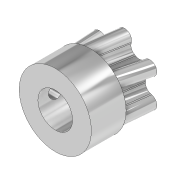
# Autodesk Inventor part: 5th Axis Drive Gear
Saved by Autodesk Inventor 2020 (Build 240168000, 168)
## iProperties
Created: 2021-06-28
Part Number: 5th Axis Drive Gear
Material: Generic
Document SubType Name: Modeling
Designer: Coy
Density: 1 g/cm^3
Appearance: Chrome - Polished
Author: Coy
Autodesk Inventor part; units mm, degrees
ref_plane "YZ Plane" through (0, 0, 0) normal (1, 0, 0) x (0, 1, 0)
ref_plane "XZ Plane" through (0, 0, 0) normal (0, 1, 0) x (-1, 0, 0)
ref_plane "XY Plane" through (0, 0, 0) normal (0, 0, 1) x (1, 0, 0)
sketch "Sketch1" plane through (0, 0, 0) normal (0, 0, 1) x (1, 0, 0)
  circle A0 centre (0, 0) radius 2.5
  circle A1 centre (0, 0) radius 5.2 construction
  line L0 (0, 0) -> (0, 5.5836) construction
  arc A2 (0.9712, 3.9619) -> (-0.9712, 3.9619) centre (0, 4.2) ccw
  line L1 (0.9221, 3.7616) -> (0.9712, 3.9619)
  line L2 (-0.9221, 3.7616) -> (-0.9712, 3.9619)
  arc A3 (-1.42, 2.6426) -> (-0.9221, 3.7616) centre (-1.8934, 3.5235) ccw
  arc A4 (0.9221, 3.7616) -> (1.42, 2.6426) centre (1.8934, 3.5235) ccw
  arc A5 (-2.9455, 2.8221) -> (-3.9167, 1.1398) centre (-3.6373, 2.1) ccw
  line L3 (-3.7187, 1.0822) -> (-3.9167, 1.1398)
  arc A6 (-2.9986, 0.0915) -> (-3.7187, 1.0822) centre (-3.9981, 0.122) ccw
  line L4 (-2.7966, 2.6794) -> (-2.9455, 2.8221)
  arc A7 (-2.7966, 2.6794) -> (-1.5786, 2.5511) centre (-2.1048, 3.4015) ccw
  arc A8 (-3.9167, -1.1398) -> (-2.9455, -2.8221) centre (-3.6373, -2.1) ccw
  line L5 (-2.7966, -2.6794) -> (-2.9455, -2.8221)
  arc A9 (-1.5786, -2.5511) -> (-2.7966, -2.6794) centre (-2.1048, -3.4015) ccw
  line L6 (-3.7187, -1.0822) -> (-3.9167, -1.1398)
  arc A10 (-3.7187, -1.0822) -> (-2.9986, -0.0915) centre (-3.9981, -0.122) ccw
  arc A11 (-0.9712, -3.9619) -> (0.9712, -3.9619) centre (0, -4.2) ccw
  line L7 (0.9221, -3.7616) -> (0.9712, -3.9619)
  arc A12 (1.42, -2.6426) -> (0.9221, -3.7616) centre (1.8934, -3.5235) ccw
  line L8 (-0.9221, -3.7616) -> (-0.9712, -3.9619)
  arc A13 (-0.9221, -3.7616) -> (-1.42, -2.6426) centre (-1.8934, -3.5235) ccw
  arc A14 (2.9455, -2.8221) -> (3.9167, -1.1398) centre (3.6373, -2.1) ccw
  line L9 (3.7187, -1.0822) -> (3.9167, -1.1398)
  arc A15 (2.9986, -0.0915) -> (3.7187, -1.0822) centre (3.9981, -0.122) ccw
  line L10 (2.7966, -2.6794) -> (2.9455, -2.8221)
  arc A16 (2.7966, -2.6794) -> (1.5786, -2.5511) centre (2.1048, -3.4015) ccw
  arc A17 (3.9167, 1.1398) -> (2.9455, 2.8221) centre (3.6373, 2.1) ccw
  line L11 (2.7966, 2.6794) -> (2.9455, 2.8221)
  arc A18 (1.5786, 2.5511) -> (2.7966, 2.6794) centre (2.1048, 3.4015) ccw
  line L12 (3.7187, 1.0822) -> (3.9167, 1.1398)
  arc A19 (3.7187, 1.0822) -> (2.9986, 0.0915) centre (3.9981, 0.122) ccw
  arc A20 (-1.42, 2.6426) -> (-1.5786, 2.5511) centre (0, 0) ccw
  arc A21 (1.5786, 2.5511) -> (1.42, 2.6426) centre (0, 0) ccw
  arc A22 (2.9986, -0.0915) -> (2.9986, 0.0915) centre (0, 0) ccw
  arc A23 (1.42, -2.6426) -> (1.5786, -2.5511) centre (0, 0) ccw
  arc A24 (-2.9986, 0.0915) -> (-2.9986, -0.0915) centre (0, 0) ccw
  arc A25 (-1.5786, -2.5511) -> (-1.42, -2.6426) centre (0, 0) ccw
  dimension "d0" = 5
  dimension "d1" = 10.4
  dimension "d3" = 2
  dimension "d4" = 2
  dimension "d5" = 2
  dimension "d8" = 360
  constraints: 48 point on circle, 26 centre point, 26 end point, 12 line through centre, 5 tangent, 2 coincident, 1 point on line, 1 vertical, 85 other
  measures "d0" diameter of A0
  measures "d1" diameter of A1
  measures "d3" diameter of A2
  measures "d4" diameter of A3
  measures "d5" diameter of A4
sketch3d "3D Sketch1"
  helix H0 starts at (2.9958, -0.0914, 0) axis through (0, 0, 0) along (0, 0, 1) pitch 166.6667 turns 0.03 hand right
sweep "Sweep1" add profiles "Sketch1" path "3D Sketch1"
sketch "Sketch2" plane through (0.787, -4.1256, 5) normal (0, 0, 1) x (0.9822873, 0.1873813, 0)
  circle A0 centre (0, 4.2) radius 2.5 projected
  arc A1 (-1.42, 6.8426) -> (-1.5786, 6.7511) centre (0, 4.2) ccw projected
  circle A2 centre (0, 4.2) radius 2.5 projected
  line L0 (-2.9455, 1.3779) -> (-2.7966, 1.5206) projected
  arc A3 (-1.5786, 1.6489) -> (-2.7966, 1.5206) centre (-2.1048, 0.7985) ccw projected
  arc A4 (-1.5786, 1.6489) -> (-1.42, 1.5574) centre (0, 4.2) ccw projected
  arc A5 (-0.9221, 0.4384) -> (-1.42, 1.5574) centre (-1.8934, 0.6765) ccw projected
  line L1 (-0.9221, 0.4384) -> (-0.9712, 0.2381) projected
  arc A6 (-0.9712, 0.2381) -> (0.9712, 0.2381) centre (0, 0) ccw projected
  line L2 (0.9712, 0.2381) -> (0.9221, 0.4384) projected
  arc A7 (1.42, 1.5574) -> (0.9221, 0.4384) centre (1.8934, 0.6765) ccw projected
  arc A8 (1.42, 1.5574) -> (1.5786, 1.6489) centre (0, 4.2) ccw projected
  arc A9 (2.7966, 1.5206) -> (1.5786, 1.6489) centre (2.1048, 0.7985) ccw projected
  line L3 (2.7966, 1.5206) -> (2.9455, 1.3779) projected
  arc A10 (2.9455, 1.3779) -> (3.9167, 3.0602) centre (3.6373, 2.1) ccw projected
  line L4 (3.9167, 3.0602) -> (3.7187, 3.1178) projected
  arc A11 (2.9986, 4.1085) -> (3.7187, 3.1178) centre (3.9981, 4.078) ccw projected
  arc A12 (2.9986, 4.1085) -> (2.9986, 4.2915) centre (0, 4.2) ccw projected
  arc A13 (3.7187, 5.2822) -> (2.9986, 4.2915) centre (3.9981, 4.322) ccw projected
  line L5 (3.7187, 5.2822) -> (3.9167, 5.3398) projected
  arc A14 (3.9167, 5.3398) -> (2.9455, 7.0221) centre (3.6373, 6.3) ccw projected
  line L6 (2.9455, 7.0221) -> (2.7966, 6.8794) projected
  arc A15 (1.5786, 6.7511) -> (2.7966, 6.8794) centre (2.1048, 7.6015) ccw projected
  arc A16 (1.5786, 6.7511) -> (1.42, 6.8426) centre (0, 4.2) ccw projected
  arc A17 (0.9221, 7.9616) -> (1.42, 6.8426) centre (1.8934, 7.7235) ccw projected
  line L7 (0.9221, 7.9616) -> (0.9712, 8.1619) projected
  arc A18 (0.9712, 8.1619) -> (-0.9712, 8.1619) centre (0, 8.4) ccw projected
  line L8 (-0.9712, 8.1619) -> (-0.9221, 7.9616) projected
  arc A19 (-1.42, 6.8426) -> (-0.9221, 7.9616) centre (-1.8934, 7.7235) ccw projected
  arc A20 (-1.42, 6.8426) -> (-1.5786, 6.7511) centre (0, 4.2) ccw projected
  arc A21 (-2.7966, 6.8794) -> (-1.5786, 6.7511) centre (-2.1048, 7.6015) ccw projected
  line L9 (-2.7966, 6.8794) -> (-2.9455, 7.0221) projected
  arc A22 (-2.9455, 7.0221) -> (-3.9167, 5.3398) centre (-3.6373, 6.3) ccw projected
  line L10 (-3.9167, 5.3398) -> (-3.7187, 5.2822) projected
  arc A23 (-2.9986, 4.2915) -> (-3.7187, 5.2822) centre (-3.9981, 4.322) ccw projected
  arc A24 (-2.9986, 4.2915) -> (-2.9986, 4.1085) centre (0, 4.2) ccw projected
  arc A25 (-3.7187, 3.1178) -> (-2.9986, 4.1085) centre (-3.9981, 4.078) ccw projected
  line L11 (-3.7187, 3.1178) -> (-3.9167, 3.0602) projected
  arc A26 (-3.9167, 3.0602) -> (-2.9455, 1.3779) centre (-3.6373, 2.1) ccw projected
  circle A27 centre (0, 4.2) radius 5.2
  point P0 (0, 4.2)
  point P1 (2.5, 4.2)
  point P2 (2.5, 4.2)
  constraints: 2 horizontal alignment, 1 centre point, 1 coincident
extrude "Extrusion1" add sketch "Sketch2" along normal blind 5
sketch "Sketch3" plane through (0, 0, 0) normal (1, 0, 0) x (0, 1, 0)
  line L0 (5.2, 5) -> (5.2, 10) projected
  line L1 (5.2, 7.5) -> (-5.2, 7.5) construction
  line L2 (-5.2, 5) -> (-5.2, 10) construction
  circle A0 centre (0, 7.5) radius 1
  point P0 (0, 0)
  dimension "d18" = 2
  constraints: 3 midpoint, 2 end point, 1 centre point
  measures "d18" diameter of A0
extrude "Extrusion2" cut sketch "Sketch3" against normal through all
body "Solid1"
